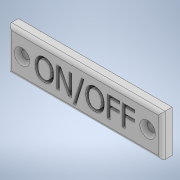
# Autodesk Inventor part: onOffSign
Saved by Autodesk Inventor 2021.2 (Build 252289000, 289)
## iProperties
Created: 2021-01-17
Part Number: onOffSign
Material: Generic
Document SubType Name: Modeling
Designer: robst
Density: 1 g/cm^3
Appearance: Default
Author: robst
Autodesk Inventor part; units mm, degrees
ref_plane "YZ Plane" through (0, 0, 0) normal (1, 0, 0) x (0, 1, 0)
ref_plane "XZ Plane" through (0, 0, 0) normal (0, 1, 0) x (-1, 0, 0)
ref_plane "XY Plane" through (0, 0, 0) normal (0, 0, 1) x (1, 0, 0)
sketch "Sketch1" plane through (0, 0, 0) normal (0, 0, 1) x (1, 0, 0)
  line L0 (-34.925, -9.525) -> (34.925, -9.525)
  line L1 (34.925, -9.525) -> (34.925, 9.525)
  line L2 (34.925, 9.525) -> (-34.925, 9.525)
  line L3 (-34.925, 9.525) -> (-34.925, -9.525)
  line L4 (-34.925, -9.525) -> (34.925, 9.525) construction
  line L5 (34.925, -9.525) -> (-34.925, 9.525) construction
  point P0 (0, 0)
  dimension "d0" = 69.85
  dimension "d1" = 19.05
  constraints: 12 end point, 2 midpoint, 2 parallel, 1 horizontal, 1 perpendicular
  measures "d0" distance of L0.start L0.end
  measures "d1" distance of L1.end L0.end
extrude "Extrusion1" add sketch "Sketch1" against normal blind 4.7625
sketch "Sketch2" plane through (0, 0, 0) normal (0, 0, 1) x (1, 0, 0)
  line L0 (-34.925, -9.525) -> (-34.925, 9.525) construction
  line L1 (-34.925, 0) -> (34.925, 0) construction
  line L2 (34.925, 9.525) -> (34.925, -9.525) construction
  spline S0 degree 2 poles (-15.2755, 3.6741) (-14.7352, 3.0412) (-14.1331, 1.1887) (-14.1331, 0) knots 0 0 0 1 2 2 2
  spline S1 degree 2 poles (-14.1331, 0) (-14.1331, -1.1578) (-14.7198, -3.0335) (-15.2755, -3.6664) knots 0 0 0 1 2 2 2
  spline S2 degree 2 poles (-15.2755, -3.6664) (-15.8621, -4.3302) (-17.4136, -4.9632) (-18.3476, -4.9632) knots 0 0 0 1 2 2 2
  spline S3 degree 2 poles (-18.3476, -4.9632) (-19.3124, -4.9632) (-20.8562, -4.3071) (-21.4197, -3.6664) knots 0 0 0 1 2 2 2
  spline S4 degree 2 poles (-21.4197, -3.6664) (-21.9677, -3.0335) (-22.5543, -1.1733) (-22.5543, 0) knots 0 0 0 1 2 2 2
  spline S5 degree 2 poles (-22.5543, 0) (-22.5543, 1.1964) (-21.96, 3.0181) (-21.412, 3.6741) knots 0 0 0 1 2 2 2
  spline S6 degree 2 poles (-21.412, 3.6741) (-20.8562, 4.3071) (-19.3047, 4.9632) (-18.3476, 4.9632) knots 0 0 0 1 2 2 2
  spline S7 degree 2 poles (-18.3476, 4.9632) (-17.375, 4.9632) (-15.8158, 4.2839) (-15.2755, 3.6741) knots 0 0 0 1 2 2 2
  spline S8 degree 2 poles (-15.453, 0) (-15.453, 0.9417) (-15.8621, 2.4005) (-16.2326, 2.8791) knots 0 0 0 1 2 2 2
  spline S9 degree 2 poles (-16.2326, 2.8791) (-16.6109, 3.3731) (-17.6761, 3.8671) (-18.3399, 3.8671) knots 0 0 0 1 2 2 2
  spline S10 degree 2 poles (-18.3399, 3.8671) (-19.0268, 3.8671) (-20.0612, 3.3886) (-20.4548, 2.8791) knots 0 0 0 1 2 2 2
  spline S11 degree 2 poles (-20.4548, 2.8791) (-20.833, 2.3928) (-21.2344, 0.9263) (-21.2344, 0) knots 0 0 0 1 2 2 2
  spline S12 degree 2 poles (-21.2344, 0) (-21.2344, -1.8757) (-19.6598, -3.8671) (-18.3399, -3.8671) knots 0 0 0 1 2 2 2
  spline S13 degree 2 poles (-18.3399, -3.8671) (-17.02, -3.8671) (-15.453, -1.8757) (-15.453, 0) knots 0 0 0 1 2 2 2
  line L3 (-5.928, -4.7625) -> (-7.3483, -4.7625)
  line L4 (-7.3483, -4.7625) -> (-11.5628, 3.4503)
  line L5 (-11.5628, 3.4503) -> (-11.5628, -4.7625)
  line L6 (-11.5628, -4.7625) -> (-12.7437, -4.7625)
  line L7 (-12.7437, -4.7625) -> (-12.7437, 4.7625)
  line L8 (-12.7437, 4.7625) -> (-10.9453, 4.7625)
  line L9 (-10.9453, 4.7625) -> (-7.109, -2.7788)
  line L10 (-7.109, -2.7788) -> (-7.109, 4.7625)
  line L11 (-7.109, 4.7625) -> (-5.928, 4.7625)
  line L12 (-5.928, 4.7625) -> (-5.928, -4.7625)
  line L13 (-0.3088, 5.187) -> (-4.0369, -6.8311)
  line L14 (-4.0369, -6.8311) -> (-5.1176, -6.8311)
  line L15 (-5.1176, -6.8311) -> (-1.4048, 5.187)
  line L16 (-1.4048, 5.187) -> (-0.3088, 5.187)
  spline S14 degree 2 poles (7.7497, 3.6741) (8.29, 3.0412) (8.8921, 1.1887) (8.8921, 0) knots 0 0 0 1 2 2 2
  spline S15 degree 2 poles (8.8921, 0) (8.8921, -1.1578) (8.3054, -3.0335) (7.7497, -3.6664) knots 0 0 0 1 2 2 2
  spline S16 degree 2 poles (7.7497, -3.6664) (7.163, -4.3302) (5.6116, -4.9632) (4.6776, -4.9632) knots 0 0 0 1 2 2 2
  spline S17 degree 2 poles (4.6776, -4.9632) (3.7127, -4.9632) (2.169, -4.3071) (1.6055, -3.6664) knots 0 0 0 1 2 2 2
  spline S18 degree 2 poles (1.6055, -3.6664) (1.0575, -3.0335) (0.4708, -1.1733) (0.4708, 0) knots 0 0 0 1 2 2 2
  spline S19 degree 2 poles (0.4708, 0) (0.4708, 1.1964) (1.0652, 3.0181) (1.6132, 3.6741) knots 0 0 0 1 2 2 2
  spline S20 degree 2 poles (1.6132, 3.6741) (2.169, 4.3071) (3.7205, 4.9632) (4.6776, 4.9632) knots 0 0 0 1 2 2 2
  spline S21 degree 2 poles (4.6776, 4.9632) (5.6502, 4.9632) (7.2094, 4.2839) (7.7497, 3.6741) knots 0 0 0 1 2 2 2
  spline S22 degree 2 poles (7.5721, 0) (7.5721, 0.9417) (7.163, 2.4005) (6.7925, 2.8791) knots 0 0 0 1 2 2 2
  spline S23 degree 2 poles (6.7925, 2.8791) (6.4143, 3.3731) (5.3491, 3.8671) (4.6853, 3.8671) knots 0 0 0 1 2 2 2
  spline S24 degree 2 poles (4.6853, 3.8671) (3.9983, 3.8671) (2.964, 3.3886) (2.5704, 2.8791) knots 0 0 0 1 2 2 2
  spline S25 degree 2 poles (2.5704, 2.8791) (2.1921, 2.3928) (1.7908, 0.9263) (1.7908, 0) knots 0 0 0 1 2 2 2
  spline S26 degree 2 poles (1.7908, 0) (1.7908, -1.8757) (3.3654, -3.8671) (4.6853, -3.8671) knots 0 0 0 1 2 2 2
  spline S27 degree 2 poles (4.6853, -3.8671) (6.0052, -3.8671) (7.5721, -1.8757) (7.5721, 0) knots 0 0 0 1 2 2 2
  line L17 (15.9779, 3.6356) -> (11.5473, 3.6356)
  line L18 (11.5473, 3.6356) -> (11.5473, 0.9494)
  line L19 (11.5473, 0.9494) -> (15.7927, 0.9494)
  line L20 (15.7927, 0.9494) -> (15.7927, -0.1775)
  line L21 (15.7927, -0.1775) -> (11.5473, -0.1775)
  line L22 (11.5473, -0.1775) -> (11.5473, -4.7625)
  line L23 (11.5473, -4.7625) -> (10.2814, -4.7625)
  line L24 (10.2814, -4.7625) -> (10.2814, 4.7625)
  line L25 (10.2814, 4.7625) -> (15.9779, 4.7625)
  line L26 (15.9779, 4.7625) -> (15.9779, 3.6356)
  line L27 (22.8091, 3.6356) -> (18.3785, 3.6356)
  line L28 (18.3785, 3.6356) -> (18.3785, 0.9494)
  line L29 (18.3785, 0.9494) -> (22.6238, 0.9494)
  line L30 (22.6238, 0.9494) -> (22.6238, -0.1775)
  line L31 (22.6238, -0.1775) -> (18.3785, -0.1775)
  line L32 (18.3785, -0.1775) -> (18.3785, -4.7625)
  line L33 (18.3785, -4.7625) -> (17.1126, -4.7625)
  line L34 (17.1126, -4.7625) -> (17.1126, 4.7625)
  line L35 (17.1126, 4.7625) -> (22.8091, 4.7625)
  line L36 (22.8091, 4.7625) -> (22.8091, 3.6356)
  point P0 (0, 0)
  constraints: 2 end point, 2 midpoint, 1 horizontal
sketch "Sketch3" plane through (0, 0, 0) normal (0, 0, 1) x (1, 0, 0)
  line L0 (-34.925, 9.525) -> (-34.925, -9.525) projected
  line L1 (34.925, -9.525) -> (34.925, 9.525) projected
  point P0 (0, 0)
  point P1 (-28.575, 0)
  point P2 (28.575, 0)
  dimension "d4" = 6.35
  dimension "d5" = 6.35
  measures "d4" distance from line of point (-28.575, 0) L0
  measures "d5" distance from line of point (28.575, 0) L1
hole "Hole1" at (-28.575, 0, 0) at (28.575, 0, 0) direction (0, 0, -1) diameter 3.81 end through all countersink diameter 7.0866 countersink angle 82 clearance for "Flat Head Machine Screw (82)" size "#6" standard "Ansi Unified Screw Threads"
extrude "Extrusion2" cut sketch "Sketch2" against normal blind 3.175
fillet "Fillet1" radius 1.5875 4 edges at (0, 9.525, 0) (34.925, 0, 0) (0, -9.525, 0) (-34.925, 0, 0)
equation "\"d0\" = width"
equation "\"d1\" = height"
equation "\"d2\" = depth"
equation "\"d4\" = edgeToHole"
equation "\"d5\" = edgeToHole"
equation "\"d13\" = textDepth"
equation "\"width\" = 69.85"
equation "\"height\" = 19.05"
equation "\"depth\" = 4.7625"
equation "\"edgeToHole\" = 6.35"
equation "\"textDepth\" = 0.666667 * depth"
body "Solid1"
